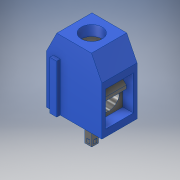
# Autodesk Inventor part: Schraubklemme_Blau_300V_16A
Saved by Autodesk Inventor 2017 SP1 (Build 210196100, 196)
## iProperties
Part Number: Schraubklemme_Blau_300V_16A
Material: Generisch
Document SubType Name: Modeling
Designer: Alex
Density: 1 g/cm^3
Appearance: Vorgabe
Author: Alex
Autodesk Inventor part; units mm, degrees
ref_plane "YZ Plane" through (0, 0, 0) normal (1, 0, 0) x (0, 1, 0)
ref_plane "XZ Plane" through (0, 0, 0) normal (0, 1, 0) x (-1, 0, 0)
sketch "Skizze4" plane through (0, 0, 0) normal (0, 1, 0) x (-1, 0, 0)
  line L0 (0, 0) -> (8, 0)
  line L1 (8, 0) -> (8, 7)
  line L2 (0, 0) -> (0, 7)
  line L3 (6.5, 10) -> (1.5, 10)
  line L4 (0, 7) -> (1.5, 10)
  line L5 (6.5, 10) -> (8, 7)
  dimension "d4" = 8
  dimension "d5" = 5
  dimension "d6" = 10
  dimension "d7" = 1.5
  constraints: 12 end point, 2 horizontal, 1 perpendicular, 1 vertical
  measures "d4" distance of L0.start L0.end
  measures "d5" distance of L3.start L3.end
  measures "d6" distance between parallel lines of L0 L3
  measures "d7" distance from line of L2 L3.end
extrude "Extrusion2" add sketch "Skizze4" along normal blind 5.08
sketch "Skizze5" plane through (0, 0, 0) normal (0, -1, 0) x (1, 0, 0)
  line L0 (-7, 0) -> (-6, 0)
  line L1 (-6, 0) -> (-6, 7)
  line L2 (-6, 7) -> (-7, 7)
  line L3 (-7, 7) -> (-7, 0)
  line L4 (0, 0) -> (-8, 0) projected
  line L5 (-8, 0) -> (-8, 7) projected
  dimension "d10" = 7
  dimension "d11" = 1
  dimension "d12" = 1
  constraints: 8 end point, 2 parallel, 1 collinear, 1 horizontal, 1 perpendicular
  measures "d10" distance of L0.end L1.end
  measures "d11" distance of L1.end L2.end
  measures "d12" distance between parallel lines of L5 L3
extrude "Extrusion3" add sketch "Skizze5" along normal blind 0.5
sketch "Skizze6" plane through (0, 5.08, 0) normal (0, 1, 0) x (1, 0, 0)
  line L0 (-7, 0) -> (-7, -7) projected
  line L1 (-7, 0) -> (-6, 0) projected
  line L2 (-6, -7) -> (-6, 0) projected
  line L3 (-7, -7) -> (-6, -7) projected
  line L4 (-6, -7) -> (-7, -7)
  line L5 (-7, -7) -> (-7, 0)
  line L6 (-7, 0) -> (-6, 0)
  line L7 (-6, 0) -> (-6, -7)
  point P0 (0, 0)
  constraints: 8 end point, 2 parallel, 1 horizontal, 1 perpendicular
extrude "Extrusion4" cut sketch "Skizze6" against normal blind 0.5
sketch "Skizze7" plane through (0, 0, 7) normal (1, 0, 0) x (0, 0, -1)
  line L0 (1, 0.54) -> (6, 0.54)
  line L1 (6, 0.54) -> (6, 4.54)
  line L2 (6, 4.54) -> (1, 4.54)
  line L3 (1, 4.54) -> (1, 0.54)
  line L4 (0, 0) -> (7, 0) projected
  line L5 (7, 0) -> (7, 5.08) projected
  dimension "d17" = 5
  dimension "d18" = 4
  dimension "d19" = 0.54
  dimension "d20" = 1
  constraints: 8 end point, 2 parallel, 1 horizontal, 1 perpendicular
  measures "d17" distance of L2.end L1.end
  measures "d18" distance of L1.end L0.end
  measures "d19" distance between parallel lines of L4 L0
  measures "d20" distance between parallel lines of L5 L1
extrude "Extrusion5" cut sketch "Skizze7" against normal blind 1.5
sketch "Skizze8" plane through (-1.5, 0, 7) normal (1, 0, 0) x (0, 0, -1)
  circle A0 centre (4, 2.54) radius 1.5
  line L0 (1, 4.54) -> (6, 4.54) projected
  line L1 (6, 4.54) -> (6, 0.54) projected
  point P0 (7, 0)
  dimension "d23" = 3
  dimension "d24" = 2
  dimension "d25" = 2
  constraints: 1 centre point
  measures "d23" diameter of A0
  measures "d24" distance from line of L0 A0.centre
  measures "d25" distance from line of L1 A0.centre
extrude "Extrusion6" cut sketch "Skizze8" against normal blind 4
sketch "Skizze10" plane through (-5.5, 2.54, 3) normal (1, 0, 0) x (0, 0, -1)
  line L0 (-2.5, -1.5) -> (-0.5, -1.5)
  line L1 (-0.5, -1.5) -> (-0.5, 1.5)
  line L2 (-0.5, 1.5) -> (-2.5, 1.5)
  line L3 (-2.5, 1.5) -> (-2.5, -1.5)
  line L4 (2, 2) -> (2, -2) projected
  line L5 (-3, 2) -> (2, 2) projected
  point P0 (3, -2.54)
  dimension "d28" = 2
  dimension "d34" = 2.5
  dimension "d41" = 0.5
  dimension "d42" = 3
  constraints: 8 end point, 2 parallel, 1 horizontal, 1 perpendicular
  measures "d28" distance of L2.end L1.end
  measures "d34" distance between parallel lines of L4 L1
  measures "d41" distance between parallel lines of L5 L2
  measures "d42" distance of L0.end L1.end
extrude "Extrusion7" add sketch "Skizze10" along normal blind 5
chamfer "Fase2" distance 0.5 angle 45 1 edges at (-0.5, 2.54, 3.5)
chamfer "Fase3" distance 1 angle 45 1 edges at (-0.5, 2.54, 5.5)
sketch "Skizze11" plane through (-6.5, 0, 10) normal (0, 0, 1) x (1, 0, 0)
  circle A0 centre (2.5, 2.54) radius 1.5
  line L0 (0, 5.08) -> (5, 5.08) projected
  line L1 (6.5, 0) -> (6.5, 5.08) projected
  line L2 (0, 0) -> (5, 0) projected
  dimension "d43" = 3
  dimension "d45" = 4
  dimension "d54" = 2.54
  constraints: 1 centre point
  measures "d43" diameter of A0
  measures "d45" distance from line of L1 A0.centre
  measures "d54" distance from line of L2 A0.centre
extrude "Extrusion8" cut sketch "Skizze11" against normal blind 1.5
sketch "Skizze12" plane through (-4, 2.54, 8.5) normal (0, 0, 1) x (1, 0, 0)
  line L0 (0.7826, 1.0062) -> (-0.3354, -1.2298)
  line L1 (-0.3354, -1.2298) -> (-0.7826, -1.0062)
  line L2 (-0.7826, -1.0062) -> (0.3354, 1.2298)
  line L3 (0.3354, 1.2298) -> (0.7826, 1.0062)
  line L4 (-0.3354, -1.2298) -> (0.3354, 1.2298) construction
  line L5 (-0.7826, -1.0062) -> (0.7826, 1.0062) construction
  line L6 (-2.5, 2.54) -> (2.5, 2.54) projected
  line L7 (4, -2.54) -> (4, 2.54) projected
  line L8 (-2.5, -2.54) -> (2.5, -2.54) projected
  point P0 (0, 0)
  point P1 (0, 0)
  point P2 (0, 0)
  dimension "d48" = 2.5
  dimension "d49" = 0.5
  dimension "d51" = 4
  dimension "d55" = 2.54
  constraints: 12 end point, 2 midpoint, 2 perpendicular, 1 coincident, 1 parallel
  measures "d48" distance of L0.start L0.end
  measures "d49" distance of L0.end L1.end
  measures "d51" distance from line of L7 point (0, 0)
  measures "d55" distance from line of L8 point (0, 0)
extrude "Extrusion9" cut sketch "Skizze12" against normal blind 0.5
sketch "Skizze14" plane through (0, 0, 0) normal (0, 0, -1) x (-1, 0, 0)
  line L0 (4.5, 2.04) -> (3.5, 2.04)
  line L1 (3.5, 2.04) -> (3.5, 3.04)
  line L2 (3.5, 3.04) -> (4.5, 3.04)
  line L3 (4.5, 3.04) -> (4.5, 2.04)
  line L4 (0, 0) -> (6, 0) projected
  line L5 (0, 0) -> (0, 5.08) projected
  dimension "d56" = 1
  dimension "d57" = 1
  dimension "d58" = 2.04
  dimension "d59" = 3.5
  constraints: 8 end point, 2 parallel, 1 horizontal, 1 perpendicular
  measures "d56" distance of L1.end L2.end
  measures "d57" distance of L0.end L1.end
  measures "d58" distance between parallel lines of L4 L0
  measures "d59" distance between parallel lines of L5 L1
extrude "Extrusion10" add sketch "Skizze14" along normal blind 4
chamfer "Fase4" distance 0.25 angle 45 4 edges at (-3.5, 2.54, -4) (-4, 2.04, -4) (-4.5, 2.54, -4) (-4, 3.04, -4)
ref_plane "Arbeitsebene1" through (0, 0, -3.5) normal (0, 0, -1) x (-1, 0, 0)
sketch "Skizze15" plane through (0, 0, -3.5) normal (0, 0, -1) x (-1, 0, 0)
  circle A0 centre (4, 2.54) radius 0.55
  line L0 (3.5, 3.04) -> (3.5, 2.04) projected
  line L1 (3.5, 3.04) -> (4.5, 3.04) projected
  point P0 (0, 0)
  dimension "d66" = 1.1
  dimension "d67" = 0.5
  dimension "d68" = 0.5
  constraints: 1 centre point
  measures "d66" diameter of A0
  measures "d67" distance from line of L0 A0.centre
  measures "d68" distance from line of L1 A0.centre
extrude "Extrusion11" add sketch "Skizze15" against normal blind 0.5 contours A0 L0 L1 | L1 A0 | A0 L0 picked at (4.1108, 2.456)
